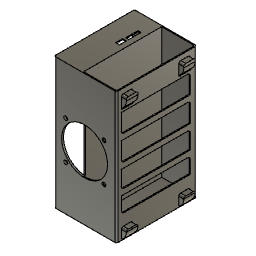
boitier alim mobo v5 (Autodesk Fusion 360 design; units mm, degrees)
Autodesk Fusion 360 part; units mm, degrees
note: some values were not read from the file. Set by a fixed rule: which sketch regions a step uses.
sketch "Esquisse1" plane through (0, 0, 0) normal (0, 0, 1) x (1, 0, 0)
  line L0 (0, 0) -> (44, 0)
  line L1 (44, 0) -> (44, 102)
  line L2 (44, 102) -> (0, 102)
  line L3 (0, 102) -> (0, 0)
  line L4 (0, 0) -> (1, 0)
  line L5 (1, 1) -> (1, 0)
  dimension "d1" = 44
  dimension "d2" = 102
  constraint horizontal L0
  constraint vertical L1
  constraint horizontal L2
  constraint vertical L3
  constraint coincident L0.start L3.end
  constraint coincident L0 L4.end
  constraint perpendicular L0 L5
  measures "d1" distance of L0.start L0.end
  measures "d2" distance of L0.start L2.end
extrude "Extrusion1" add sketch "Esquisse1" along normal blind 1 makes body 1
sketch "Esquisse2" plane through (0, 0, 1) normal (0, 0, 1) x (-1, 0, 0)
  line L0 (0, 0) -> (-44, 0)
  line L1 (-44, 0) -> (-44, -102)
  line L2 (-44, -102) -> (0, -102)
  line L3 (0, -102) -> (0, 0)
  line L4 (-1, -1) -> (-43, -1)
  line L5 (-43, -1) -> (-43, -101)
  line L6 (-43, -101) -> (-1, -101)
  line L7 (-1, -101) -> (-1, -1)
  dimension "d5" = 42
  dimension "d6" = 100
  constraint horizontal L4
  constraint vertical L5
  constraint horizontal L6
  constraint vertical L7
  measures "d5" distance of L4.start L4.end
  measures "d6" distance of L4.start L6.end
extrude "Extrusion2" add sketch "Esquisse2" along normal blind 170 bodies 1
sketch "Esquisse3" plane through (44, 0, 0) normal (1, 0, 0) x (0, 1, 0)
  line L0 (0, 0) -> (102, 0)
  line L1 (102, 0) -> (102, 171)
  line L2 (102, 171) -> (0, 171)
  line L3 (0, 171) -> (0, 0)
  line L4 (15, 135) -> (85, 135)
  line L5 (85, 135) -> (85, 45)
  line L6 (85, 45) -> (15, 45)
  line L7 (15, 45) -> (15, 135)
  constraint horizontal L4
  constraint vertical L5
  constraint horizontal L6
  constraint vertical L7
extrude "Extrusion3" cut sketch "Esquisse3" against normal blind 1 contours L4 L5 L6 L7 bodies 1
extrude "Extrusion4" add 1 faces at (0, 68, 57) along direction (-1, 0, 0) blind 1 on bodies 1 bodies 1
sketch "Esquisse4" plane through (-1, 0, 0) normal (-1, 0, 0) x (0, -1, 0)
  line L0 (-102, 0) -> (0, 0)
  line L1 (0, 0) -> (0, 171)
  line L2 (0, 171) -> (-102, 171)
  line L3 (-102, 171) -> (-102, 0)
  line L4 (-1, 1) -> (-101, 1)
  line L5 (-101, 1) -> (-101, 170)
  line L6 (-101, 170) -> (-1, 170)
  line L7 (-1, 170) -> (-1, 1)
  constraint horizontal L4
  constraint vertical L5
  constraint horizontal L6
  constraint vertical L7
extrude "Extrusion5" add sketch "Esquisse4" along normal blind 35 bodies 1
sketch "Esquisse10" plane through (0, 0, 1) normal (0, 0, 1) x (-1, 0, 0)
  line L0 (-1, -1) -> (-43, -1)
  line L1 (-43, -1) -> (-43, -101)
  line L2 (-43, -101) -> (-1, -101)
  line L3 (-1, -101) -> (-1, -1)
  circle A0 centre (-34, -10) radius 2.6531
extrude "Extrusion10" cut sketch "Esquisse10" against normal blind 10 contours A0 bodies 1
sketch "Esquisse12" plane through (44, 0, 0) normal (1, 0, 0) x (0, 1, 0)
  line L0 (85, 135) -> (85, 45)
  line L1 (85, 45) -> (15, 45)
  line L2 (15, 45) -> (15, 135)
  line L3 (15, 135) -> (85, 135)
  line L4 (0, 0) -> (102, 0)
  line L5 (102, 0) -> (102, 171)
  line L6 (102, 171) -> (0, 171)
  line L7 (0, 171) -> (0, 0)
  line L8 (5, 165) -> (20, 165)
  line L9 (20, 165) -> (20, 155)
  line L10 (20, 155) -> (5, 155)
  line L11 (5, 155) -> (5, 165)
  line L12 (95, 5) -> (80, 5)
  line L13 (80, 5) -> (80, 15)
  line L14 (80, 15) -> (95, 15)
  line L15 (95, 15) -> (95, 5)
  line L16 (95, 155) -> (80, 155)
  line L17 (80, 155) -> (80, 165)
  line L18 (80, 165) -> (95, 165)
  line L19 (95, 165) -> (95, 155)
  line L20 (20, 5) -> (5, 5)
  line L21 (5, 5) -> (5, 15)
  line L22 (5, 15) -> (20, 15)
  line L23 (20, 15) -> (20, 5)
  constraint horizontal L8
  constraint vertical L9
  constraint horizontal L10
  constraint vertical L11
  constraint horizontal L14
  constraint vertical L15
  constraint horizontal L12
  constraint vertical L13
  constraint horizontal L18
  constraint vertical L19
  constraint horizontal L16
  constraint vertical L17
  constraint horizontal L22
  constraint vertical L23
  constraint horizontal L20
  constraint vertical L21
extrude "Extrusion12" add sketch "Esquisse12" along normal blind 8 contours L8 L9 L10 L11 | L12 L13 L14 L15 | L16 L17 L18 L19 | L20 L21 L22 L23 bodies 1
fillet "Congé1" radius 15 4 edges at (44, 12.5, 5) (44, 87.5, 5) (44, 87.5, 155) (44, 12.5, 155) on bodies 1
fillet "Congé2" radius 12.5 4 edges at (52, 12.5, 155) (52, 87.5, 155) (52, 87.5, 5) (52, 12.5, 5) on bodies 1
extrude "Extrusion14" add 1 faces at (17.3333, 102, 114) along direction (0, 1, 0) blind 0.4 on bodies 1 bodies 1
move_face "DécalerLesFaces1" offset 0.4 1 faces at (-9.3333, 0, 114) on bodies 1
move_face "DécalerLesFaces2" offset 0.4 1 faces at (-23.6667, 34.3333, 171) on bodies 1
extrude "Extrusion15" add 1 faces at (17.3333, -0.4, 114.2667) along direction (0, -1, 0) blind 1 on bodies 1 bodies 1
extrude "Extrusion16" cut 1 faces at (29, 1, 114.6) along direction (0, -1, 0) blind 1 on bodies 1 bodies 1
extrude "Extrusion17" add 1 faces at (-9.3333, 102.4, 57.1333) along direction (0, 1, 0) blind 1 on bodies 1 bodies 1
extrude "Extrusion18" cut 1 faces at (15, 101, 114.6) along direction (0, 1, 0) blind 1 on bodies 1 bodies 1
extrude "Extrusion20" add 1 faces at (44, 40, 35) along direction (1, 0, 0) blind 1.4 on bodies 1 bodies 1
extrude "Extrusion21" cut 1 faces at (43, 62.3333, 15.6667) along direction (1, 0, 0) blind 1 on bodies 1 bodies 1
sketch "Esquisse15" plane through (0, 0, 0) normal (0, 0, -1) x (1, 0, 0)
  circle A0 centre (34, -10) radius 2.6531
  line L0 (-36, 1.4) -> (-36, -103.4)
  line L1 (-36, -103.4) -> (45.4, -103.4)
  line L2 (45.4, -103.4) -> (45.4, -95)
  line L3 (45.4, -95) -> (44, -95)
  line L4 (44, -95) -> (44, -80)
  line L5 (44, -80) -> (45.4, -80)
  line L6 (45.4, -80) -> (45.4, -20)
  line L7 (45.4, -20) -> (44, -20)
  line L8 (44, -20) -> (44, -5)
  line L9 (44, -5) -> (45.4, -5)
  line L10 (45.4, -5) -> (45.4, 1.4)
  line L11 (45.4, 1.4) -> (-36, 1.4)
  circle A1 centre (34, -10) radius 4.0799
  constraint concentric A0 A1
extrude "Extrusion22" cut sketch "Esquisse15" against normal blind 5 contours A1 bodies 1
sketch "Esquisse16" plane through (0, 103.4, 0) normal (0, 1, 0) x (-1, 0, 0)
  line L0 (-45.4, 0) -> (36, 0)
  line L1 (36, 0) -> (36, 171.4)
  line L2 (36, 171.4) -> (-45.4, 171.4)
  line L3 (-45.4, 171.4) -> (-45.4, 0)
  line L4 (-30.6547, 110.3782) -> (19.3453, 110.3782)
  line L5 (19.3453, 110.3782) -> (19.3453, 60.3782)
  line L6 (19.3453, 60.3782) -> (-30.6547, 60.3782)
  line L7 (-30.6547, 60.3782) -> (-30.6547, 110.3782)
  circle A0 centre (19.3453, 110.3782) radius 2.5
  circle A1 centre (-30.6547, 110.3782) radius 2.5
  circle A2 centre (-30.6547, 60.3782) radius 2.5
  circle A3 centre (19.3453, 60.3782) radius 2.5
  dimension "d67" = 50
  dimension "d68" = 50
  dimension "d69" = 5
  dimension "d70" = 5
  dimension "d71" = 5
  dimension "d72" = 5
  constraint horizontal L4
  constraint vertical L5
  constraint horizontal L6
  constraint vertical L7
  constraint coincident L4.end L5.start
  constraint coincident L4.start L7.end
  constraint coincident L6.end L7.start
  constraint coincident L5.end L6.start
  measures "d67" distance of L4.start L4.end
  measures "d68" distance of L4.start L6.end
  measures "d69" diameter of A0
  measures "d70" diameter of A1
  measures "d71" diameter of A2
  measures "d72" diameter of A3
sketch "Esquisse18" plane through (0, 103.4, 0) normal (0, 1, 0) x (-1, 0, 0)
  line L0 (-45.4, 0) -> (36, 0)
  line L1 (36, 0) -> (36, 171.4)
  line L2 (36, 171.4) -> (-45.4, 171.4)
  line L3 (-45.4, 171.4) -> (-45.4, 0)
  circle A0 centre (-5, 85) radius 30
sketch "Esquisse19" plane through (0, -1.4, 0) normal (0, -1, 0) x (1, 0, 0)
  line L0 (-36, 0) -> (45.4, 0)
  line L1 (45.4, 0) -> (45.4, 171.4)
  line L2 (45.4, 171.4) -> (-36, 171.4)
  line L3 (-36, 171.4) -> (-36, 0)
  circle A0 centre (3.7054, 83.2966) radius 30
  line L4 (-20.9924, 108.5115) -> (29.0076, 108.5115)
  line L5 (29.0076, 108.5115) -> (29.0076, 58.5115)
  line L6 (29.0076, 58.5115) -> (-20.9924, 58.5115)
  line L7 (-20.9924, 58.5115) -> (-20.9924, 108.5115)
  circle A1 centre (29.0076, 108.5115) radius 2.5
  circle A2 centre (-20.9924, 108.5115) radius 2.5
  circle A3 centre (-20.9924, 58.5115) radius 2.5
  circle A4 centre (29.0076, 58.5115) radius 2.5
  dimension "d103" = 60
  dimension "d104" = 50
  dimension "d105" = 50
  dimension "d106" = 5
  dimension "d107" = 5
  dimension "d108" = 5
  dimension "d109" = 5
  constraint horizontal L4
  constraint vertical L5
  constraint horizontal L6
  constraint vertical L7
  constraint coincident L4.end L5.start
  constraint coincident L4.start L7.end
  constraint coincident L6.end L7.start
  constraint coincident L5.end L6.start
  measures "d103" diameter of A0
  measures "d104" distance of L4.start L4.end
  measures "d105" distance of L4.start L6.end
  measures "d106" diameter of A1
  measures "d107" diameter of A2
  measures "d108" diameter of A3
  measures "d109" diameter of A4
extrude "Extrusion38" cut sketch "Esquisse19" against normal blind 3 contours A0 L5 | A0 L4 L5 L6 L7 | A0 L4 | L4 L5 A1 | L4 L5 A1 | A0 L6 | L5 L6 A4 | L5 L6 A4 | A0 L7 | L4 L7 A2 | L4 L7 A2 | L6 L7 A3 | L6 L7 A3 bodies 1
sketch "Esquisse20" plane through (0, -1.4, 0) normal (0, -1, 0) x (1, 0, 0)
  circle A0 centre (29.0076, 108.5115) radius 2.5
  circle A1 centre (29.0076, 58.5115) radius 2.5
  circle A2 centre (-20.9924, 58.5115) radius 2.5
  circle A3 centre (3.7054, 83.2966) radius 30
  circle A4 centre (-20.9924, 108.5115) radius 2.5
  line L0 (-36, 0) -> (45.4, 0)
  line L1 (45.4, 0) -> (45.4, 171.4)
  line L2 (45.4, 171.4) -> (-36, 171.4)
  line L3 (-36, 171.4) -> (-36, 0)
  circle A5 centre (-25, 160) radius 5
  dimension "d112" = 10
  measures "d112" diameter of A5
sketch "Esquisse21" plane through (0, -1.4, 0) normal (0, -1, 0) x (1, 0, 0)
sketch "Esquisse22" plane through (0, -1.4, 0) normal (0, -1, 0) x (1, 0, 0)
  circle A0 centre (29.0076, 108.5115) radius 2.5
  circle A1 centre (29.0076, 58.5115) radius 2.5
  circle A2 centre (-20.9924, 58.5115) radius 2.5
  circle A3 centre (3.7054, 83.2966) radius 30
  circle A4 centre (-20.9924, 108.5115) radius 2.5
  line L0 (-36, 0) -> (45.4, 0)
  line L1 (45.4, 0) -> (45.4, 171.4)
  line L2 (45.4, 171.4) -> (-36, 171.4)
  line L3 (-36, 171.4) -> (-36, 0)
extrude "Extrusion41" add 1 faces at (44.5193, 95, 142.4568) along direction (0, -1, 0) blind 15 on bodies 1 bodies 1
extrude "Extrusion42" add 1 faces at (44.5193, 20, 142.4568) along direction (0, -1, 0) blind 15 on bodies 1 bodies 1
extrude "Extrusion43" add 1 faces at (44.9185, 95, 0.505) along direction (0, -1, 0) blind 15 on bodies 1 bodies 1
extrude "Extrusion44" add 1 faces at (44.9185, 20, 0.505) along direction (0, -1, 0) blind 15 on bodies 1 bodies 1
extrude "Extrusion45" cut 1 faces at (44.4667, 61.6667, 45) along direction (0, 0, -1) blind 15 on bodies 1 bodies 1
extrude "Extrusion46" cut 1 faces at (44.4667, 15, 100) along direction (0, -1, 0) blind 10 on bodies 1 bodies 1
extrude "Extrusion47" cut 1 faces at (44.4667, 85, 65) along direction (0, 1, 0) blind 10 on bodies 1 bodies 1
extrude "Extrusion48" cut 1 faces at (44.4667, 35, 135) along direction (0, 0, 1) blind 10 on bodies 1 bodies 1
sketch "Esquisse23" plane through (0, 5, 0) normal (0, 1, 0) x (-1, 0, 0)
  line L0 (-44, 30) -> (-44, 145)
  line L1 (-44, 145) -> (-45.4, 145)
  line L2 (-45.4, 145) -> (-45.4, 30)
  line L3 (-45.4, 30) -> (-44, 30)
  line L4 (-45.4, 87.5) -> (-44, 87.5)
  line L5 (-45.4, 145) -> (-45.4, 115)
  line L6 (-45.4, 87.5) -> (-45.4, 57.5)
  line L7 (-45.4, 57.5) -> (-44, 57.5)
  line L8 (-44, 57.5) -> (-44, 50.5)
  line L9 (-44, 50.5) -> (-45.4, 50.5)
  line L10 (-45.4, 50.5) -> (-45.4, 57.5)
  line L11 (-45.4, 87.5) -> (-44, 87.5)
  line L12 (-44, 87.5) -> (-44, 80.5)
  line L13 (-44, 80.5) -> (-45.4, 80.5)
  line L14 (-45.4, 80.5) -> (-45.4, 87.5)
  line L15 (-45.4, 115) -> (-44, 115)
  line L16 (-44, 115) -> (-44, 108)
  line L17 (-44, 108) -> (-45.4, 108)
  line L18 (-45.4, 108) -> (-45.4, 115)
  dimension "d135" = 30
  dimension "d136" = 7
  dimension "d137" = 7
  dimension "d138" = 7
  constraint midpoint L2 L4.start
  constraint midpoint L0 L4.end
  constraint coincident L1.end L2.start
  constraint coincident L2 L5.end
  constraint perpendicular L1 L5
  constraint perpendicular L4 L6
  constraint horizontal L7
  constraint vertical L8
  constraint horizontal L9
  constraint vertical L10
  constraint horizontal L11
  constraint vertical L12
  constraint horizontal L13
  constraint vertical L14
  constraint horizontal L15
  constraint vertical L16
  constraint horizontal L17
  constraint vertical L18
  measures "d135" distance of L4.start L6.end
  measures "d136" distance of L6.end L9.end
  measures "d137" distance of L4.start L13.end
  measures "d138" distance of L5.end L17.end
extrude "Extrusion49" add sketch "Esquisse23" along normal blind 90 contours L0 L2 L7 L8 L9 L10 | L0 L2 L4 L6 L11 L12 L13 L14 | L0 L2 L15 L16 L17 L18 bodies 1
extrude "Extrusion50" add 1 faces at (44.4667, 35, 115) along direction (0, 0, 1) blind 5 on bodies 1 bodies 1
extrude "Extrusion51" cut 1 faces at (44.9333, 35, 108) along direction (0, 0, 1) blind 5 on bodies 1 bodies 1
fillet "Congé3" radius 3.5 3 edges at (44.7, 95, 113) (44.7, 95, 80.5) (44.7, 95, 50.5) on bodies 1
fillet "Congé4" radius 3.5 3 edges at (44.7, 5, 57.5) (44.7, 5, 87.5) (44.7, 5, 120) on bodies 1
fillet "Congé5" radius 3.5 1 edges at (44.7, 95, 145) on bodies 1
fillet "Congé6" radius 3.5 1 edges at (44.7, 5, 30) on bodies 1
fillet "Congé7" radius 2 2 edges at (44, 0, 86.2) (44, 102, 86.2) on bodies 1
fillet "Congé8" radius 2 2 edges at (45.4, -1.4, 85.7) (45.4, 103.4, 85.7) on bodies 1
fillet "Congé9" radius 2.5 4 edges at (48.7, 95, 165) (48.7, 80, 165) (48.7, 20, 165) (48.7, 5, 165) on bodies 1
fillet "Congé10" radius 2.5 4 edges at (48.7, 95, 15) (48.7, 80, 15) (48.7, 20, 15) (48.7, 5, 15) on bodies 1
sketch "Esquisse24" plane through (0, 101, 0) normal (0, -1, 0) x (1, 0, 0)
  line L0 (-1, 1) -> (-1, 170)
  line L1 (-1, 170) -> (-36, 170)
  line L2 (-36, 170) -> (-36, 1)
  line L3 (-36, 1) -> (-1, 1)
  line L4 (-36, 170) -> (-34, 170)
  line L5 (-34, 170) -> (-24, 170)
  line L6 (-24, 170) -> (-24, 160)
  line L7 (-24, 160) -> (-34, 160)
  line L8 (-34, 160) -> (-34, 170)
  line L9 (-36, 1) -> (-34, 1)
  line L10 (-34, 1) -> (-24, 1)
  line L11 (-24, 1) -> (-24, 11)
  line L12 (-24, 11) -> (-34, 11)
  line L13 (-34, 11) -> (-34, 1)
  dimension "d161" = 10
  dimension "d162" = 10
  dimension "d163" = 2
  dimension "d164" = 10
  dimension "d165" = 10
  constraint coincident L1.end L2.start
  constraint coincident L1 L4.end
  constraint perpendicular L2 L4
  constraint horizontal L5
  constraint vertical L6
  constraint horizontal L7
  constraint vertical L8
  constraint coincident L2.end L3.start
  constraint perpendicular L2 L9
  constraint horizontal L10
  constraint vertical L11
  constraint horizontal L12
  constraint vertical L13
  measures "d161" distance of L4.end L5.end
  measures "d162" distance of L4.end L7.end
  measures "d163" distance of L2.end L9.end
  measures "d164" distance of L9.end L10.end
  measures "d165" distance of L9.end L12.end
extrude "Extrusion52" add sketch "Esquisse24" along normal blind 10 contours L3 L10 L11 L12 L13 | L1 L5 L6 L7 L8 bodies 1
fillet "Congé11" radius 5 3 edges at (-29, 91, 160) (-29, 101, 160) (-29, 91, 170) on bodies 1
sketch "Esquisse25" plane through (0, 1, 0) normal (0, 1, 0) x (-1, 0, 0)
  arc A0 (1, 53.6679) -> (1, 112.9253) centre (-3.7054, 83.2966) ccw
  line L0 (1, 53.6679) -> (1, 1)
  line L1 (1, 1) -> (36, 1)
  line L2 (36, 1) -> (36, 170)
  line L3 (36, 170) -> (1, 170)
  line L4 (1, 170) -> (1, 112.9253)
  circle A1 centre (20.9924, 58.5115) radius 2.5
  circle A2 centre (20.9924, 108.5115) radius 2.5
  line L5 (36, 1) -> (34, 1)
  line L6 (34, 1) -> (24, 1)
  line L7 (24, 1) -> (24, 11)
  line L8 (24, 11) -> (34, 11)
  line L9 (34, 11) -> (34, 1)
  line L10 (36, 170) -> (34, 170)
  line L11 (34, 170) -> (24, 170)
  line L12 (24, 170) -> (24, 160)
  line L13 (24, 160) -> (34, 160)
  line L14 (34, 160) -> (34, 170)
  dimension "d170" = 2
  dimension "d171" = 10
  dimension "d172" = 10
  dimension "d173" = 2
  dimension "d174" = 10
  dimension "d175" = 10
  constraint coincident L1.end L2.start
  constraint horizontal L5
  constraint horizontal L6
  constraint vertical L7
  constraint horizontal L8
  constraint vertical L9
  constraint coincident L2.end L3.start
  constraint horizontal L10
  constraint horizontal L11
  constraint vertical L12
  constraint horizontal L13
  constraint vertical L14
  measures "d170" distance of L1.end L5.end
  measures "d171" distance of L5.end L6.end
  measures "d172" distance of L5.end L8.end
  measures "d173" distance of L2.end L10.end
  measures "d174" distance of L10.end L11.end
  measures "d175" distance of L10.end L13.end
extrude "Extrusion53" add sketch "Esquisse25" along normal blind 10 contours L1 L6 L7 L8 L9 | L3 L11 L12 L13 L14 bodies 1
fillet "Congé12" radius 5 9 edges at (-29, 11, 1) (-29, 11, 11) (-29, 1, 11) (-29, 11, 160) (-29, 1, 160) (-29, 11, 170) (-29, 91, 1) (-29, 91, 11) (-29, 101, 11) on bodies 1
sketch "Esquisse26" plane through (-34, 0, 0) normal (-1, 0, 0) x (0, -1, 0)
  arc A0 (-11, 165) -> (-6, 160) centre (-6, 165) ccw
  arc A1 (-1, 155) -> (-6, 160) centre (-6, 155) ccw
  line L0 (-1, 155) -> (-1, 170)
  line L1 (-1, 170) -> (-16, 170)
  arc A2 (-11, 165) -> (-16, 170) centre (-16, 165) ccw
  circle A3 centre (-6, 165) radius 1.5
  dimension "d180" = 3
  constraint concentric A0 A3
  measures "d180" diameter of A3
extrude "Extrusion54" cut sketch "Esquisse26" against normal blind 10 contours A3 bodies 1
sketch "Esquisse27" plane through (-34, 0, 0) normal (-1, 0, 0) x (0, -1, 0)
  arc A0 (-96, 160) -> (-91, 165) centre (-96, 165) ccw
  arc A1 (-86, 170) -> (-91, 165) centre (-86, 165) ccw
  line L0 (-86, 170) -> (-101, 170)
  line L1 (-101, 170) -> (-101, 155)
  arc A2 (-96, 160) -> (-101, 155) centre (-96, 155) ccw
  circle A3 centre (-96, 165) radius 1.5
  dimension "d183" = 3
  constraint concentric A0 A3
  measures "d183" diameter of A3
extrude "Extrusion55" cut sketch "Esquisse27" against normal blind 10 contours A3 bodies 1
sketch "Esquisse28" plane through (-34, 0, 0) normal (-1, 0, 0) x (0, -1, 0)
  arc A0 (-91, 6) -> (-96, 11) centre (-96, 6) ccw
  arc A1 (-101, 16) -> (-96, 11) centre (-96, 16) ccw
  line L0 (-101, 16) -> (-101, 1)
  line L1 (-101, 1) -> (-86, 1)
  arc A2 (-91, 6) -> (-86, 1) centre (-86, 6) ccw
  circle A3 centre (-96, 6) radius 1.5
  dimension "d186" = 3
  constraint concentric A0 A3
  measures "d186" diameter of A3
extrude "Extrusion56" cut sketch "Esquisse28" against normal blind 10 contours A3 bodies 1
sketch "Esquisse29" plane through (-34, 0, 0) normal (-1, 0, 0) x (0, -1, 0)
  arc A0 (-6, 11) -> (-11, 6) centre (-6, 6) ccw
  arc A1 (-16, 1) -> (-11, 6) centre (-16, 6) ccw
  line L0 (-16, 1) -> (-1, 1)
  line L1 (-1, 1) -> (-1, 16)
  arc A2 (-6, 11) -> (-1, 16) centre (-6, 16) ccw
  circle A3 centre (-6, 6) radius 1.5
  dimension "d189" = 3
  constraint concentric A0 A3
  measures "d189" diameter of A3
extrude "Extrusion57" cut sketch "Esquisse29" against normal blind 10 contours A3 bodies 1
sketch "Esquisse30" plane through (-1, 0, 0) normal (-1, 0, 0) x (0, -1, 0)
  line L0 (-1, 53.6679) -> (-1.6, 53.6679)
  line L1 (-1.6, 53.6679) -> (-1.6, 112.9253)
  line L2 (-1.6, 112.9253) -> (-1, 112.9253)
  line L3 (-1, 112.9253) -> (-1, 170)
  line L4 (-1, 170) -> (-101, 170)
  line L5 (-101, 170) -> (-101, 1)
  line L6 (-101, 1) -> (-1, 1)
  line L7 (-1, 1) -> (-1, 53.6679)
  circle A0 centre (-29.8921, 8.0021) radius 5.2844
extrude "Extrusion58" cut sketch "Esquisse30" against normal blind 10 contours A0 bodies 1
sketch "Esquisse31" plane through (-1, 0, 0) normal (-1, 0, 0) x (0, -1, 0)
  circle A0 centre (-29.8921, 8.0021) radius 5.2844
  line L0 (-1, 53.6679) -> (-1.6, 53.6679)
  line L1 (-1.6, 53.6679) -> (-1.6, 112.9253)
  line L2 (-1.6, 112.9253) -> (-1, 112.9253)
  line L3 (-1, 112.9253) -> (-1, 170)
  line L4 (-1, 170) -> (-101, 170)
  line L5 (-101, 170) -> (-101, 1)
  line L6 (-101, 1) -> (-1, 1)
  line L7 (-1, 1) -> (-1, 53.6679)
  line L8 (-85, 170) -> (-15, 170)
  line L9 (-15, 170) -> (-15, 70)
  line L10 (-15, 70) -> (-85, 70)
  line L11 (-85, 70) -> (-85, 170)
  line L12 (-85, 170) -> (-82, 170)
  line L13 (-82, 170) -> (-82, 151)
  line L14 (-82, 151) -> (-85, 151)
  line L15 (-85, 151) -> (-85, 170)
  circle A1 centre (-82, 151) radius 3
  line L16 (-85, 170) -> (-18, 170)
  line L17 (-18, 170) -> (-18, 167)
  line L18 (-18, 167) -> (-85, 167)
  line L19 (-85, 167) -> (-85, 170)
  circle A2 centre (-18, 167) radius 3
  line L20 (-85, 170) -> (-44, 170)
  line L21 (-44, 170) -> (-44, 104)
  line L22 (-44, 104) -> (-85, 104)
  line L23 (-85, 104) -> (-85, 170)
  circle A3 centre (-44, 104) radius 3
  line L24 (-85, 167) -> (-82, 167)
  line L25 (-82, 167) -> (-82, 86)
  line L26 (-82, 86) -> (-85, 86)
  line L27 (-85, 86) -> (-85, 167)
  circle A4 centre (-82, 86) radius 3
  line L28 (-85, 170) -> (-47, 170)
  line L29 (-47, 170) -> (-47, 72)
  line L30 (-47, 72) -> (-85, 72)
  line L31 (-85, 72) -> (-85, 170)
  circle A5 centre (-47, 72) radius 3
  dimension "d194" = 70
  dimension "d195" = 100
  dimension "d196" = 3
  dimension "d197" = 19
  dimension "d198" = 6
  dimension "d199" = 67
  dimension "d200" = 3
  dimension "d201" = 6
  dimension "d202" = 41
  dimension "d203" = 66
  dimension "d204" = 6
  dimension "d205" = 3
  dimension "d206" = 81
  dimension "d207" = 6
  dimension "d208" = 38
  dimension "d209" = 98
  dimension "d210" = 6
  constraint horizontal L8
  constraint vertical L9
  constraint horizontal L10
  constraint vertical L11
  constraint coincident L4 L8.start
  constraint horizontal L12
  constraint vertical L13
  constraint horizontal L14
  constraint vertical L15
  constraint coincident L13.end L14.start
  constraint horizontal L16
  constraint vertical L17
  constraint horizontal L18
  constraint vertical L19
  constraint coincident L17.end L18.start
  constraint horizontal L20
  constraint vertical L21
  constraint horizontal L22
  constraint vertical L23
  constraint coincident L21.end L22.start
  constraint horizontal L24
  constraint vertical L25
  constraint horizontal L26
  constraint vertical L27
  constraint coincident L25.end L26.start
  constraint horizontal L28
  constraint vertical L29
  constraint horizontal L30
  constraint vertical L31
  constraint coincident L29.end L30.start
  measures "d194" distance of L8.start L8.end
  measures "d195" distance of L8.start L10.end
  measures "d196" distance of L8.start L12.end
  measures "d197" distance of L8.start L14.end
  measures "d198" diameter of A1
  measures "d199" distance of L8.start L16.end
  measures "d200" distance of L8.start L18.end
  measures "d201" diameter of A2
  measures "d202" distance of L8.start L20.end
  measures "d203" distance of L8.start L22.end
  measures "d204" diameter of A3
  measures "d205" distance of L18.end L24.end
  measures "d206" distance of L18.end L26.end
  measures "d207" diameter of A4
  measures "d208" distance of L8.start L28.end
  measures "d209" distance of L8.start L30.end
  measures "d210" diameter of A5
extrude "Extrusion59" add sketch "Esquisse31" along normal blind 5 separate body contours L17 L18 A2 | L17 L18 A2 | L13 L14 A1 L25 | L14 A1 L25 | L13 A1 L25 | L10 A5 | L10 L29 L30 A5 | L21 L22 A3 | L21 L22 A3 | L25 L26 A4 | L25 L26 A4 | L29 L30 A5 makes body 2 at (-4.3333, 79.3653, 84.5652) makes body 3 at (-4.3333, 20.7644, 165.8347) makes body 4 at (-4.3333, 41.2356, 105.1653) makes body 5 at (-4.3333, 80.2488, 148.5642) makes body 6 at (-2.6667, 49.8191, 70.9739)
sketch "Esquisse32" plane through (-6, 0, 0) normal (-1, 0, 0) x (0, -1, 0)
  circle A0 centre (-18, 167) radius 3
  circle A1 centre (-18, 167) radius 1.5
  dimension "d213" = 3
  constraint concentric A0 A1
  measures "d213" diameter of A1
extrude "Extrusion60" cut sketch "Esquisse32" against normal blind 6 contours A1 bodies 1 3
sketch "Esquisse33" plane through (-6, 0, 0) normal (-1, 0, 0) x (0, -1, 0)
  circle A0 centre (-82, 151) radius 3
  circle A1 centre (-82, 151) radius 1.5
  dimension "d216" = 3
  constraint concentric A0 A1
  measures "d216" diameter of A1
extrude "Extrusion61" cut sketch "Esquisse33" against normal blind 6 contours A1 bodies 1 5
sketch "Esquisse34" plane through (-6, 0, 0) normal (-1, 0, 0) x (0, -1, 0)
  circle A0 centre (-44, 104) radius 3
  circle A1 centre (-44, 104) radius 1.5
  dimension "d219" = 3
  constraint concentric A0 A1
  measures "d219" diameter of A1
extrude "Extrusion62" cut sketch "Esquisse34" against normal blind 6 contours A1 bodies 1 4
sketch "Esquisse35" plane through (-6, 0, 0) normal (-1, 0, 0) x (0, -1, 0)
  circle A0 centre (-82, 86) radius 3
  circle A1 centre (-82, 86) radius 1.5
  dimension "d222" = 3
  constraint concentric A0 A1
  measures "d222" diameter of A1
extrude "Extrusion63" cut sketch "Esquisse35" against normal blind 6 contours A1 bodies 1 2
sketch "Esquisse36" plane through (-6, 0, 0) normal (-1, 0, 0) x (0, -1, 0)
  circle A0 centre (-47, 72) radius 3
  circle A1 centre (-47, 72) radius 1.5
  dimension "d225" = 3
  constraint concentric A0 A1
  measures "d225" diameter of A1
extrude "Extrusion64" cut sketch "Esquisse36" against normal blind 6 contours A1 bodies 1 6
fillet "Congé13" radius 2 2 edges at (-36, 103.4, 85.7) (-36, -1.4, 85.7) on bodies 1
sketch "Esquisse37" plane through (0, 101, 0) normal (0, -1, 0) x (1, 0, 0)
  line L0 (-24, 16) -> (-24, 1)
  line L1 (-24, 1) -> (-1, 1)
  line L2 (-1, 1) -> (-1, 170)
  line L3 (-1, 170) -> (-24, 170)
  line L4 (-24, 170) -> (-24, 155)
  line L5 (-24, 155) -> (-34, 155)
  line L6 (-34, 155) -> (-34, 170)
  line L7 (-34, 170) -> (-36, 170)
  line L8 (-36, 170) -> (-36, 1)
  line L9 (-36, 1) -> (-34, 1)
  line L10 (-34, 1) -> (-34, 16)
  line L11 (-34, 16) -> (-24, 16)
  line L12 (-10, 15) -> (-20, 15)
  line L13 (-20, 15) -> (-20, 30)
  line L14 (-20, 30) -> (-10, 30)
  line L15 (-10, 30) -> (-10, 15)
  constraint horizontal L12
  constraint vertical L13
  constraint horizontal L14
  constraint vertical L15
extrude "Extrusion65" cut sketch "Esquisse37" against normal blind 14 contours L12 L13 L14 L15 bodies 1
fillet "Congé14" radius 3 4 edges at (-20, 102.2, 30) (-20, 102.2, 15) (-10, 102.2, 15) (-10, 102.2, 30) on bodies 1
fillet "Congé15" radius 1 2 edges at (1, 1.6, 83.2966) (-1, 1.6, 83.2966) on bodies 1
sketch "Esquisse38" plane through (0, 0, 170) normal (0, 0, -1) x (1, 0, 0)
  line L0 (-34, -16) -> (-34, -1)
  line L1 (-34, -1) -> (-36, -1)
  line L2 (-36, -1) -> (-36, -101)
  line L3 (-36, -101) -> (-34, -101)
  line L4 (-34, -101) -> (-34, -86)
  line L5 (-34, -86) -> (-24, -86)
  line L6 (-24, -86) -> (-24, -101)
  line L7 (-24, -101) -> (-1, -101)
  line L8 (-1, -101) -> (-1, -1)
  line L9 (-1, -1) -> (-24, -1)
  line L10 (-24, -1) -> (-24, -16)
  line L11 (-24, -16) -> (-34, -16)
  line L12 (-1, -85) -> (-6, -85)
  line L13 (-6, -85) -> (-6, -15)
  line L14 (-6, -15) -> (-1, -15)
  line L15 (-1, -15) -> (-1, -85)
  line L16 (-6, -85) -> (-6, -82)
  line L17 (-6, -82) -> (-10, -82)
  line L18 (-10, -82) -> (-10, -66)
  line L19 (-10, -66) -> (-6, -66)
  line L20 (-6, -66) -> (-6, -82)
  line L21 (-6, -85) -> (-6, -63)
  line L22 (-6, -63) -> (-11, -63)
  line L23 (-11, -63) -> (-11, -54)
  line L24 (-11, -54) -> (-6, -54)
  line L25 (-6, -54) -> (-6, -63)
  dimension "d236" = 5
  dimension "d237" = 70
  dimension "d238" = 4
  dimension "d239" = 16
  dimension "d240" = 22
  dimension "d241" = 5
  dimension "d242" = 9
  constraint coincident L8 L12.start
  constraint horizontal L12
  constraint vertical L13
  constraint horizontal L14
  constraint vertical L15
  constraint coincident L13 L16.end
  constraint horizontal L17
  constraint vertical L18
  constraint horizontal L19
  constraint vertical L20
  constraint perpendicular L17 L21
  constraint horizontal L22
  constraint vertical L23
  constraint horizontal L24
  constraint vertical L25
  measures "d236" distance of L12.start L12.end
  measures "d237" distance of L12.start L14.end
  measures "d238" distance of L16.end L17.end
  measures "d239" distance of L16.end L19.end
  measures "d240" distance of L12.end L21.end
  measures "d241" distance of L21.end L22.end
  measures "d242" distance of L21.end L24.end
extrude "Extrusion66" cut sketch "Esquisse38" against normal blind 10 contours L13 L22 L23 L24 L25 | L13 L17 L18 L19 L20 L21 bodies 1
